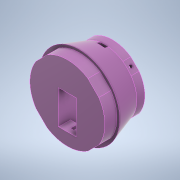
# Autodesk Inventor part: Case
Saved by Autodesk Inventor 2022.2 (Build 262287010, 287A)
## iProperties
Created: 2022-02-16
Part Number: Case
Material: ABS Plastic
Document SubType Name: Modeling
Designer: smiku
Density: 1.06 g/cm^3
Appearance: Smooth - Purple
Author: smiku
Autodesk Inventor part; units mm, degrees
ref_plane "YZ Plane" through (0, 0, 0) normal (1, 0, 0) x (0, 1, 0)
ref_plane "XZ Plane" through (0, 0, 0) normal (0, 1, 0) x (-1, 0, 0)
ref_plane "XY Plane" through (0, 0, 0) normal (0, 0, 1) x (1, 0, 0)
sketch "Sketch1" plane through (0, 0, 0) normal (0, 0, 1) x (1, 0, 0)
  line L0 (-19.2384, -29.2384) -> (19.2384, -29.2384) construction
  line L1 (29.2384, -19.2384) -> (29.2384, 19.2384) construction
  line L2 (19.2384, 29.2384) -> (-19.2384, 29.2384) construction
  line L3 (-29.2384, 19.2384) -> (-29.2384, -19.2384) construction
  line L4 (-29.2384, -29.2384) -> (29.2384, 29.2384) construction
  line L5 (29.2384, -29.2384) -> (-29.2384, 29.2384) construction
  line L6 (-29.2384, 19.2384) -> (-19.2384, 29.2384) construction
  line L7 (19.2384, 29.2384) -> (29.2384, 19.2384) construction
  line L8 (29.2384, -19.2384) -> (19.2384, -29.2384) construction
  line L9 (-19.2384, -29.2384) -> (-29.2384, -19.2384) construction
  circle A0 centre (0, 0) radius 35 construction
  line L10 (-19.4455, 29.7384) -> (-29.7384, 19.4455)
  line L11 (-29.7384, 19.4455) -> (-29.7384, -19.4455) construction
  line L12 (-29.7384, -19.4455) -> (-19.4455, -29.7384)
  line L13 (-19.4455, -29.7384) -> (19.4455, -29.7384) construction
  line L14 (19.4455, -29.7384) -> (29.7384, -19.4455)
  line L15 (29.7384, -19.4455) -> (29.7384, 19.4455) construction
  line L16 (29.7384, 19.4455) -> (19.4455, 29.7384)
  line L17 (19.4455, 29.7384) -> (-19.4455, 29.7384) construction
  line L18 (22.6657, 32.9586) -> (32.9586, 22.6657)
  line L19 (19.4455, 29.7384) -> (22.6657, 32.9586) construction
  line L20 (29.7384, 19.4455) -> (32.9586, 22.6657) construction
  line L21 (29.7384, -19.4455) -> (19.4455, -29.7384) construction
  line L22 (19.4455, -29.7384) -> (22.6657, -32.9586) construction
  line L23 (22.6657, -32.9586) -> (32.9586, -22.6657)
  line L24 (32.9586, -22.6657) -> (29.7384, -19.4455) construction
  arc A1 (32.9586, -22.6657) -> (32.9586, 22.6657) centre (0, 0) ccw
  line L25 (-29.7384, -19.4455) -> (-19.4455, -29.7384) construction
  line L26 (-19.4455, -29.7384) -> (-22.6657, -32.9586) construction
  line L27 (-22.6657, -32.9586) -> (-32.9586, -22.6657)
  line L28 (-32.9586, -22.6657) -> (-29.7384, -19.4455) construction
  arc A2 (-22.6657, -32.9586) -> (22.6657, -32.9586) centre (0, 0) ccw
  line L29 (-19.4455, 29.7384) -> (-29.7384, 19.4455) construction
  line L30 (-29.7384, 19.4455) -> (-32.9586, 22.6657) construction
  line L31 (-32.9586, 22.6657) -> (-22.6657, 32.9586)
  line L32 (-22.6657, 32.9586) -> (-19.4455, 29.7384) construction
  arc A3 (22.6657, 32.9586) -> (-22.6657, 32.9586) centre (0, 0) ccw
  arc A4 (-32.9586, 22.6657) -> (-32.9586, -22.6657) centre (0, 0) ccw
  arc A5 (19.4455, 29.7384) -> (-19.4455, 29.7384) centre (0, 0) ccw
  arc A6 (-29.7384, 19.4455) -> (-29.7384, -19.4455) centre (0, 0) ccw
  arc A7 (-19.4455, -29.7384) -> (19.4455, -29.7384) centre (0, 0) ccw
  arc A8 (29.7384, -19.4455) -> (29.7384, 19.4455) centre (0, 0) ccw
  dimension "d64" = 70
  dimension "d56" = 10
  dimension "d57" = 10
  dimension "d58" = 10
  dimension "d59" = 10
  dimension "d60" = 10
  dimension "d61" = 10
  dimension "d62" = 10
  dimension "d63" = 10
  dimension "d65" = 0.5
  dimension "d68" = 40
  constraints: 66 end point, 16 point on circle, 13 point on line, 12 equal length, 8 centre point, 8 perpendicular, 7 coincident, 3 midpoint, 2 concentric, 1 horizontal, 10 other
  measures "d56" distance of L3.start L5.end
  measures "d57" distance of L2.end L5.end
  measures "d58" distance of L2.start L4.end
  measures "d59" distance of L1.end L4.end
  measures "d60" distance of L1.start L5.start
  measures "d61" distance of L0.end L5.start
  measures "d62" distance of L0.start L4.start
  measures "d63" distance of L3.end L4.start
  measures "d65" distance between parallel lines of L2 L17
  measures "d68" radius of A1
extrude "Extrusion1" add sketch "Sketch1" against normal blind 10
sketch "Sketch5" plane through (32.9586, 22.6657, -10) normal (0.7071068, 0.7071068, 0) x (-0.7071068, 0.7071068, 0)
  line L0 (0, 10) -> (14.5563, 10) construction
  line L1 (0, 10) -> (0, 0) construction
  line L2 (14.5563, 0) -> (0, 0) construction
  line L3 (14.5563, 10) -> (14.5563, 0) construction
  line L4 (0, 10) -> (14.5563, 10) construction
  line L5 (0, 0) -> (14.5563, 10) construction
  circle A0 centre (7.2782, 5) radius 2
  point P0 (7.2782, 10)
  dimension "d69" = 4
  constraints: 2 end point, 1 centre point, 1 midpoint
  measures "d69" diameter of A0
extrude "Extrusion7" cut sketch "Sketch5" against normal up to next
pattern_circular "Circular Pattern1" count 4 over 360 about axis through (0, 0, -10) along (0, 0, 1) of "Extrusion7"
sketch "Sketch12" plane through (0, 0, 0) normal (0, 0, 1) x (1, 0, 0)
  line L0 (-11, -33.7861) -> (-11, 33.7861)
  line L1 (11, 33.7861) -> (11, -33.7861)
  line L2 (11, -33.7861) -> (-11, 33.7861) construction
  line L3 (-11, -33.7861) -> (11, 33.7861) construction
  circle A0 centre (0, 0) radius 40
  arc A1 (19.4455, 29.7384) -> (-19.4455, 29.7384) centre (0, 0) ccw construction
  arc A2 (-19.4455, -29.7384) -> (19.4455, -29.7384) centre (0, 0) ccw construction
  arc A3 (-19.4455, -29.7384) -> (19.4455, -29.7384) centre (0, 0) ccw construction
  arc A4 (11, 33.7861) -> (-11, 33.7861) centre (0, 0) ccw
  arc A5 (-11, -33.7861) -> (11, -33.7861) centre (0, 0) ccw
  point P0 (0, 0)
  point P1 (0, 0)
  point P2 (22.6657, 32.9586)
  dimension "d141" = 22
  constraints: 8 end point, 7 point on circle, 4 coincident, 4 midpoint, 2 centre point, 1 parallel, 1 vertical, 3 other
  measures "d141" distance of L0.end L1.start
extrude "Extrusion13" add sketch "Sketch12" along normal blind 31 contours L0 A4 L1 A5 | A0
sketch "Sketch13" plane through (0, 0, 31) normal (0, 0, 1) x (1, 0, 0)
  circle A0 centre (0, 0) radius 50
  dimension "d146" = 100
  constraints: 1 centre point, 1 coincident
  measures "d146" diameter of A0
loft "Loft2" add profiles "Sketch12", "Sketch13" contours L0 A4 L1 A5 | A0 / all
sketch "Sketch14" plane through (0, 0, 31) normal (0, 0, 1) x (1, 0, 0)
  line L0 (11, -40) -> (-11, -40)
  line L1 (-11, -40) -> (-11, 20)
  line L2 (-11, 20) -> (11, 20)
  line L3 (11, 20) -> (11, -40)
  line L4 (11, -40) -> (-11, 20) construction
  line L5 (-11, -40) -> (11, 20) construction
  point P0 (0, 0)
  point P1 (0, -10)
  point P2 (0, -10)
  point P3 (0, -10)
  dimension "d152" = 22
  dimension "d153" = 60
  dimension "d154" = 10
  constraints: 12 end point, 4 midpoint, 2 parallel, 1 horizontal, 1 perpendicular, 1 vertical alignment
  measures "d152" distance of L1.end L2.end
  measures "d153" distance of L0.end L1.end
  measures "d154" distance of point (0, -10) point (0, 0)
loft "Loft3" cut profiles "Sketch14", "Sketch12" contours all / L0 A4 L1 A5
sketch "Sketch15" plane through (0, 0, 31) normal (0, 0, 1) x (1, 0, 0)
  circle A0 centre (0, 0) radius 46.5
  line L0 (-11, -31) -> (11, -31)
  line L1 (11, -31) -> (11, 11)
  line L2 (11, 11) -> (-11, 11)
  line L3 (-11, 11) -> (-11, -31)
  line L4 (-11, -31) -> (11, 11) construction
  line L5 (11, -31) -> (-11, 11) construction
  line L6 (0, 0) -> (46.5, 0) construction
  line L7 (0, 0) -> (32.8805, 32.8805) construction
  circle A1 centre (0, 0) radius 50 construction
  line L8 (-11, -40) -> (-11, 20) construction
  line L9 (11, 20) -> (11, -40) construction
  line L10 (-11, 20) -> (11, -40) construction
  line L11 (25.391, 38.9557) -> (38.9557, 25.391)
  line L12 (-38.9557, 25.391) -> (-25.391, 38.9557)
  line L13 (-25.391, -38.9557) -> (-38.9557, -25.391)
  line L14 (38.9557, -25.391) -> (25.391, -38.9557)
  point P0 (0, -10)
  point P1 (-34.5503, 31.1211)
  point P2 (10.3254, -45.3785)
  point P3 (0, -10)
  point P4 (32.1734, 32.1734)
  point P5 (-32.1734, 32.1734)
  point P6 (-32.1734, -32.1734)
  point P7 (32.1734, -32.1734)
  dimension "d160" = 42
  dimension "d161" = 45
  dimension "d170" = 3.5
  dimension "d172" = 46.5
  dimension "d173" = 45.5
  dimension "d176" = 360
  constraints: 26 end point, 5 midpoint, 5 point on circle, 3 point on line, 2 horizontal, 2 parallel, 1 centre point, 1 coincident, 1 perpendicular, 17 other
  measures "d160" distance of L1.end L0.end
  measures "d161" angle of L7 L6
  measures "d170" radial gap between concentric circles of A1 A0
  measures "d172" distance of L11.end L6.start
  measures "d173" distance of point (32.173, 32.173) L6.start
extrude "Extrusion14" add sketch "Sketch15" along normal blind 15 contours A0 L14 L13 L12 L11
sketch "Sketch16" plane through (0, 0, 31) normal (0, 0, -1) x (-1, 0, 0)
  line L0 (-11, -31) -> (-11, -40) construction
  line L1 (11, 11) -> (-11, 11) construction
  line L2 (-11, -31) -> (11, 11) construction
  line L3 (5, 14.75) -> (-5, 14.75) construction
  line L4 (-5, 14.75) -> (-5, -34.75) construction
  line L5 (-5, -34.75) -> (5, -34.75) construction
  line L6 (5, -34.75) -> (5, 14.75) construction
  line L7 (5, 14.75) -> (-5, -34.75) construction
  line L8 (-5, 14.75) -> (5, -34.75) construction
  circle A0 centre (5, 14.75) radius 2
  circle A1 centre (-5, 14.75) radius 2
  circle A2 centre (-5, -34.75) radius 2
  circle A3 centre (5, -34.75) radius 2
  point P0 (0, 0)
  point P1 (0, -10)
  dimension "d178" = 10
  dimension "d179" = 49.5
  dimension "d180" = 4
  constraints: 14 end point, 4 centre point, 4 coincident, 3 equal radius, 3 midpoint, 2 parallel, 1 horizontal, 1 perpendicular
  measures "d178" distance of L5.end L4.end
  measures "d179" distance of L4.end L3.end
  measures "d180" diameter of A0
extrude "Extrusion15" cut sketch "Sketch16" against normal blind 10
sketch "Sketch17" plane through (0, 0, 0) normal (1, 0, 0) x (0, 1, 0)
  line L0 (50, 31) -> (40, 0) construction
  line L1 (40, 0) -> (40, -10) construction
  line L2 (40, -10) -> (35.5317, -10) construction
  line L3 (35.5317, -10) -> (35.5317, 0) construction
  line L4 (20, 31) -> (11, 31) construction
  line L5 (11, 31) -> (11, 46) construction
  line L6 (11, 46) -> (46.5, 46) construction
  line L7 (46.5, 46) -> (46.5, 31) construction
  line L8 (46.5, 31) -> (50, 31) construction
  line L9 (-40, 0) -> (-50, 31) construction
  line L10 (-50, 31) -> (-46.5, 31) construction
  line L11 (-46.5, 31) -> (-46.5, 46) construction
  line L12 (-46.5, 46) -> (-31, 46) construction
  line L13 (-31, 46) -> (-31, 31) construction
  line L14 (-31, 31) -> (-40, 31) construction
  line L15 (-35.5317, 0) -> (-35.5317, -10) construction
  line L16 (-35.5317, -10) -> (-40, -10) construction
  line L17 (-40, -10) -> (-40, 0) construction
  line L18 (11, 31) -> (20, 31)
  line L19 (20, 31) -> (11, 40)
  line L20 (11, 40) -> (11, 31)
  line L21 (-40, 31) -> (-31, 40)
  line L22 (-31, 40) -> (-31, 31)
  line L23 (-31, 31) -> (-40, 31)
  point P0 (0, 0)
  constraints: 12 end point, 3 collinear, 2 perpendicular, 2 point on line, 2 other
extrude "Extrusion16" cut sketch "Sketch17" along normal mid plane 4
sketch "Sketch18" plane through (-11, 11, 46) normal (0, -1, 0) x (1, 0, 0)
  line L0 (16, -41) -> (6, -41)
  line L1 (6, -41) -> (6, -46)
  line L2 (6, -46) -> (16, -46)
  line L3 (16, -46) -> (16, -41)
  point P0 (11, -46)
  point P1 (11, -46)
  dimension "d185" = 10
  dimension "d186" = 5
  constraints: 8 end point, 2 parallel, 1 coincident, 1 horizontal, 1 midpoint, 1 perpendicular
  measures "d185" distance of L2.end L1.end
  measures "d186" distance of L1.end L0.end
extrude "Extrusion17" cut sketch "Sketch18" against normal through all
equation "\"d57\" = d56"
equation "\"d58\" = d56"
equation "\"d59\" = d58"
equation "\"d60\" = d56"
equation "\"d61\" = d60"
equation "\"d62\" = d56"
equation "\"d63\" = d62"
body "Solid1"
